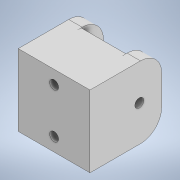
# Autodesk Inventor part: Bearing_Holder
Saved by Autodesk Inventor 2022 (Build 260153000, 153)
## iProperties
Created: 2022-02-28
Part Number: Bearing_Holder
Material: Generic
Document SubType Name: Modeling
Designer: Mlees
Density: 1 g/cm^3
Appearance: Default
Author: Mlees
Autodesk Inventor part; units mm, degrees
ref_plane "YZ Plane" through (0, 0, 0) normal (1, 0, 0) x (0, 1, 0)
ref_plane "XZ Plane" through (0, 0, 0) normal (0, 1, 0) x (-1, 0, 0)
sketch "Sketch1" plane through (0, 0, 0) normal (0, 1, 0) x (-1, 0, 0)
  line L0 (0, 0) -> (16, 0)
  line L1 (16, 0) -> (16, -20)
  line L2 (16, -20) -> (0, -20)
  line L3 (0, -20) -> (0, 0)
  dimension "d0" = 16
  dimension "d1" = 20
  constraints: 8 end point, 3 perpendicular, 1 horizontal
  measures "d0" distance of L0.start L0.end
  measures "d1" distance of L0.end L1.end
extrude "Extrusion1" add sketch "Sketch1" along normal blind 16
ref_plane "Work Plane1" through (0, 0, -15) normal (0, 0, -1) x (-1, 0, 0)
sketch "Sketch2" plane through (0, 0, -15) normal (0, 0, -1) x (-1, 0, 0)
  line L0 (16, 16) -> (0, 16) projected
  line L1 (8, 16) -> (3, 16)
  line L2 (3, 16) -> (13, 16)
  line L3 (0, 0) -> (0, 16) projected
  line L4 (0, 8) -> (3, 8)
  line L5 (3, 8) -> (13, 8)
  line L6 (13, 8) -> (13, 16)
  line L7 (13, 16) -> (3, 16)
  line L8 (3, 16) -> (3, 8)
  dimension "d5" = 5
  constraints: 14 end point, 2 midpoint, 2 perpendicular, 1 horizontal, 1 point on line
  measures "d5" distance of L1.start L1.end
revolve "Revolution1" cut sketch "Sketch2" angle 360 about axis through (-3, 8, -15) along (-1, 0, 0) contours L6 L5 L8 L0
fillet "Fillet1" radius 4.75 4 edges at (-8, 14.245, -20) (-8, 1.755, -20) (-8, 16, -20) (-8, 0, -20)
sketch "Sketch3" plane through (-16, 0, 0) normal (0, 0, 1) x (1, 0, 0)
  line L0 (0, 16) -> (16, 16) projected
  line L1 (0, 16) -> (16, 16)
  line L2 (16, 16) -> (16, 0)
  line L3 (16, 0) -> (0, 0)
  line L4 (0, 0) -> (0, 16)
  constraints: 8 end point, 2 parallel, 1 horizontal, 1 perpendicular
extrude "Extrusion2" cut sketch "Sketch3" against normal blind 4
sketch "Sketch4" plane through (0, 4.75, -20) normal (1, 0, 0) x (0, 0, -1)
  arc A0 (-5, 11.25) -> (-5, -4.75) centre (-5, 3.25) ccw projected
  circle A1 centre (-5, 3.25) radius 1
  point P0 (-20, -4.75)
  dimension "d12" = 2
  constraints: 1 centre point, 1 coincident
  measures "d12" diameter of A1
extrude "Extrusion3" cut sketch "Sketch4" against normal up to surface (16 mm away)
sketch "Sketch5" plane through (-16, 0, -4) normal (0, 0, 1) x (1, 0, 0)
  line L0 (0, 16) -> (16, 16) projected
  circle A0 centre (8, 3) radius 1
  circle A1 centre (8, 13) radius 1
  point P0 (16, 0)
  dimension "d16" = 2
  constraints: 2 centre point
  measures "d16" diameter of A0
extrude "Extrusion4" cut sketch "Sketch5" against normal blind 10
sketch "Sketch6" plane through (0, 16, 0) normal (0, 1, 0) x (1, 0, 0)
  line L0 (-13, 15) -> (-3, 15) projected
  line L1 (-13, 16.0838) -> (-3, 16.0838) projected
  line L2 (-3, 15) -> (-13, 15)
  line L3 (-13, 15) -> (-13, 16.0838)
  line L4 (-13, 16.0838) -> (-3, 16.0838)
  line L5 (-3, 16.0838) -> (-3, 15)
  point P0 (0, 0)
  constraints: 8 end point, 2 parallel, 1 horizontal, 1 perpendicular
extrude "Extrusion5" cut sketch "Sketch6" against normal up to surface (16 mm away)
body "Solid1"
